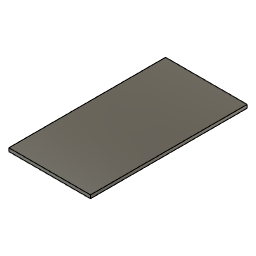
ionicthrusterassembly v7 (Autodesk Fusion 360 archive; units mm, degrees)
design "test"
Autodesk Fusion 360 part; units mm, degrees
(part 1 of 2)
sketch "Sketch1" plane through (0, 0, 0) normal (0, 0, 1) x (1, 0, 0)
  line L0 (0, 0) -> (125, 0)
  line L1 (125, 0) -> (125, 240)
  line L2 (125, 240) -> (0, 240)
  line L3 (0, 240) -> (0, 0)
  dimension "d1" = 125
  dimension "d2" = 240
  constraint horizontal L0
  constraint vertical L1
  constraint horizontal L2
  constraint vertical L3
  constraint coincident L0.start L3.end
  measures "d1" distance of L0.start L0.end
  measures "d2" distance of L0.start L2.end
extrude "Extrude1" add sketch "Sketch1" along normal blind 5

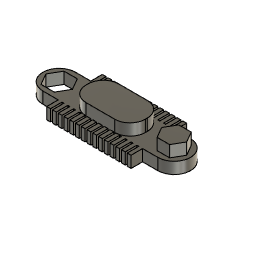
design "modularfingers"
Autodesk Fusion 360 part; units mm, degrees
sketch "Sketch1" plane through (0, 0, 0) normal (0, 0, 1) x (1, 0, 0)
  line L0 (0, -4.25) -> (30, -4.25)
  arc A0 (30, -4.25) -> (30, 4.25) centre (30, 0) ccw
  line L1 (30, 4.25) -> (0, 4.25)
  arc A1 (0, 4.25) -> (0, -4.25) centre (0, 0) ccw
  line L2 (0, 0) -> (30, 0) construction
  circle A2 centre (0, 0) radius 3 construction
  line L3 (-1.7321, 3) -> (-3.4641, 0)
  line L4 (-3.4641, 0) -> (-1.7321, -3)
  line L5 (-1.7321, -3) -> (1.7321, -3)
  line L6 (1.7321, -3) -> (3.4641, 0)
  line L7 (3.4641, 0) -> (1.7321, 3)
  line L8 (1.7321, 3) -> (-1.7321, 3)
  circle A3 centre (30, 0) radius 2.825 construction
  line L9 (33.262, 0) -> (31.631, 2.825)
  line L10 (31.631, 2.825) -> (28.369, 2.825)
  line L11 (28.369, 2.825) -> (26.738, 0)
  line L12 (26.738, 0) -> (28.369, -2.825)
  line L13 (28.369, -2.825) -> (31.631, -2.825)
  line L14 (31.631, -2.825) -> (33.262, 0)
  line L15 (18.738, -4.25) -> (11.262, -4.25)
  line L16 (7.262, -0.25) -> (7.262, 0.25)
  line L17 (11.262, 4.25) -> (18.738, 4.25)
  line L18 (22.738, 0.25) -> (22.738, -0.25)
  line L19 (22.738, -4.25) -> (7.262, 4.25) construction
  line L20 (7.262, -4.25) -> (22.738, 4.25) construction
  arc A4 (11.262, 4.25) -> (7.262, 0.25) centre (11.262, 0.25) ccw
  arc A5 (7.262, -0.25) -> (11.262, -4.25) centre (11.262, -0.25) ccw
  arc A6 (18.738, -4.25) -> (22.738, -0.25) centre (18.738, -0.25) ccw
  arc A7 (22.738, 0.25) -> (18.738, 4.25) centre (18.738, 0.25) ccw
  point P0 (30, 0)
  point P1 (15, 0)
  dimension "d1" = 30
  dimension "d2" = 4.25
  dimension "d14" = 60
  dimension "d15" = 5.65
  dimension "d16" = 6
  dimension "d17" = 60
  dimension "d18" = 4
  dimension "d19" = 4
  constraint tangent L0 A0
  constraint tangent A0 L1
  constraint parallel L0 L1
  constraint tangent L1 A1
  constraint tangent L0 A1
  constraint horizontal L2
  constraint coincident A1.centre L2.start
  constraint concentric A1 A2
  constraint concentric A0 A3
  constraint coincident P0 A0.centre
  constraint tangent A3 L9
  constraint tangent A2 L7
  constraint horizontal L15
  constraint perpendicular L15 L16
  constraint parallel L15 L17
  constraint parallel L16 L18
  constraint coincident L19 P1
  constraint coincident L20 P1
  constraint coincident L0 L19.start
  constraint midpoint L2 P1
  constraint coincident L19.end L16
  constraint coincident L19.end L17
  constraint tangent L16 A4
  constraint tangent L17 A4
  constraint coincident L20.start L16
  constraint coincident L20.start L15
  constraint tangent L16 A5
  constraint tangent L15 A5
  constraint equal A4 A5
  constraint coincident L19.start L18
  constraint coincident L19.start L15
  constraint tangent L18 A6
  constraint tangent L15 A6
  constraint equal A4 A6
  constraint coincident L20.end L18
  constraint coincident L20.end L17
  constraint tangent L18 A7
  constraint tangent L17 A7
  constraint equal A4 A7
  measures "d1" distance of A0.end L1.end
  measures "d2" radius of A0
  measures "d14" angle of L2 L7
  measures "d15" diameter of A3
  measures "d16" diameter of A2
  measures "d17" angle of L2 L14
  measures "d18" distance of L11.end L18
  measures "d19" radius of A4
extrude "Extrude1" add sketch "Sketch1" along normal blind 3 contours L0 L1 A1 L16 A4 A5 | L0 A0 L1 L18 A6 A7 makes body 1 at (4.2732, -1.6372, 0) makes body 2 at (25.8943, 1.4006, 0)
extrude "Extrude3" add sketch "Sketch1" along normal blind 6 contours L0 L1 L15 L16 L17 L18 A4 A5 A6 A7 | L9 L10 L11 L12 L13 L14 bodies 1 2
sketch "Sketch3" plane through (0, -4.25, 0) normal (0, -1, 0) x (1, 0, 0)
  line L0 (0, 0) -> (30, 0)
  line L1 (30, 0) -> (30, 3)
  line L2 (30, 3) -> (18.738, 3)
  line L3 (18.738, 3) -> (18.738, 6)
  line L4 (18.738, 6) -> (11.262, 6)
  line L5 (11.262, 6) -> (11.262, 3)
  line L6 (11.262, 3) -> (0, 3)
  line L7 (0, 3) -> (0, 0)
  line L8 (4, 3) -> (5, 3)
  line L9 (5, 3) -> (5, 0)
  line L10 (5, 0) -> (4, 0)
  line L11 (4, 0) -> (4, 3)
  line L12 (6.5, 3) -> (6.5, 0)
  line L13 (5.5, 3) -> (6.5, 3)
  line L14 (5.5, 0) -> (5.5, 3)
  line L15 (6.5, 0) -> (5.5, 0)
  line L16 (8, 3) -> (8, 0)
  line L17 (7, 3) -> (8, 3)
  line L18 (7, 0) -> (7, 3)
  line L19 (8, 0) -> (7, 0)
  line L20 (9.5, 3) -> (9.5, 0)
  line L21 (8.5, 3) -> (9.5, 3)
  line L22 (8.5, 0) -> (8.5, 3)
  line L23 (9.5, 0) -> (8.5, 0)
  line L24 (11, 3) -> (11, 0)
  line L25 (10, 3) -> (11, 3)
  line L26 (10, 0) -> (10, 3)
  line L27 (11, 0) -> (10, 0)
  line L28 (12.5, 3) -> (12.5, 0)
  line L29 (11.5, 3) -> (12.5, 3)
  line L30 (11.5, 0) -> (11.5, 3)
  line L31 (12.5, 0) -> (11.5, 0)
  line L32 (14, 3) -> (14, 0)
  line L33 (13, 3) -> (14, 3)
  line L34 (13, 0) -> (13, 3)
  line L35 (14, 0) -> (13, 0)
  line L36 (15.5, 3) -> (15.5, 0)
  line L37 (14.5, 3) -> (15.5, 3)
  line L38 (14.5, 0) -> (14.5, 3)
  line L39 (15.5, 0) -> (14.5, 0)
  line L40 (17, 3) -> (17, 0)
  line L41 (16, 3) -> (17, 3)
  line L42 (16, 0) -> (16, 3)
  line L43 (17, 0) -> (16, 0)
  line L44 (18.5, 3) -> (18.5, 0)
  line L45 (17.5, 3) -> (18.5, 3)
  line L46 (17.5, 0) -> (17.5, 3)
  line L47 (18.5, 0) -> (17.5, 0)
  line L48 (20, 3) -> (20, 0)
  line L49 (19, 3) -> (20, 3)
  line L50 (19, 0) -> (19, 3)
  line L51 (20, 0) -> (19, 0)
  line L52 (21.5, 3) -> (21.5, 0)
  line L53 (20.5, 3) -> (21.5, 3)
  line L54 (20.5, 0) -> (20.5, 3)
  line L55 (21.5, 0) -> (20.5, 0)
  line L56 (23, 3) -> (23, 0)
  line L57 (22, 3) -> (23, 3)
  line L58 (22, 0) -> (22, 3)
  line L59 (23, 0) -> (22, 0)
  line L60 (24.5, 3) -> (24.5, 0)
  line L61 (23.5, 3) -> (24.5, 3)
  line L62 (23.5, 0) -> (23.5, 3)
  line L63 (24.5, 0) -> (23.5, 0)
  line L64 (26, 3) -> (26, 0)
  line L65 (25, 3) -> (26, 3)
  line L66 (25, 0) -> (25, 3)
  line L67 (26, 0) -> (25, 0)
  dimension "d39" = 1
  dimension "d40" = 4
  dimension "d47" = 21
  dimension "d48" = 0
  constraint horizontal L8
  constraint vertical L9
  constraint horizontal L10
  constraint vertical L11
  constraint coincident L0 L9.end
  constraint coincident L6 L8.start
  measures "d39" distance of L9.end L10.end
  measures "d40" distance of L7 L11
extrude "Extrude5" add sketch "Sketch3" along normal blind 3 contours L0 L6 L8 L9 L10 L11 | L0 L6 L12 L13 L14 L15 | L0 L6 L16 L17 L18 L19 | L0 L6 L20 L21 L22 L23 | L0 L6 L24 L25 L26 L27 | L0 L28 L29 L30 L31 | L0 L32 L33 L34 L35 | L0 L36 L37 L38 L39 | L0 L2 L48 L49 L50 L51 | L0 L40 L41 L42 L43 | L0 L2 L52 L53 L54 L55 | L0 L44 L45 L46 L47 | L0 L2 L56 L57 L58 L59 | L0 L2 L60 L61 L62 L63 | L0 L2 L64 L65 L66 L67 bodies 1
ref_plane "WorkPlane2" through (28, 0, 1.5) normal (0, -1, 0) x (1, 0, 0)
mirror "Mirror2" about plane through (28, 0, 1.5) normal (0, -1, 0) of bodies 1 merged
equation "d1 = length"
equation "d2 = arc_Length"
equation "height = 6 mm"
equation "length = 30 mm"
equation "total_length = 30 mm + 8.5 mm"
equation "arc_Length = ( total_length - length ) / 2"
equation "DegreePolygon = ( 360 / 6 ) * 1 deg"
equation "Polygon_Length = 6 mm"
equation "NPolygonSides = 6"
equation "d14 = DegreePolygon"
equation "d15 = Polygon_Length - Hole_OFFSET"
equation "d16 = Polygon_Length"
equation "d17 = DegreePolygon"
equation "d18 = offsetdistance"
equation "d19 = arc_Polygon"
equation "arc_Polygon = 4 mm"
equation "offsetdistance = 4 mm"
equation "d22 = ( height / 2 mm ) * 1 mm"
equation "d26 = height"
equation "Hole_OFFSET = 0.35 mm"
equation "d39 = pattounes_width"
equation "d40 = pattounes_offset"
equation "pattounes_offset = 4 mm"
equation "pattounes_width = 1 mm"
equation "NPattounes = 15"
equation "d45 = NPattounes"
equation "d47 = length - pattounes_offset * 2 - pattounes_width"
equation "d51 = -arc_Length"

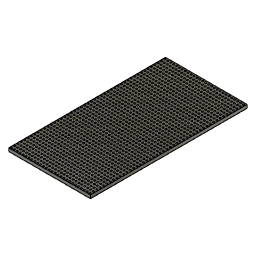
design "base"
Autodesk Fusion 360 part; units mm, degrees
sketch "Sketch1" plane through (0, 0, 0) normal (0, 0, 1) x (1, 0, 0)
  line L0 (0, 0) -> (125, 0)
  line L1 (125, 0) -> (125, 240)
  line L2 (125, 240) -> (0, 240)
  line L3 (0, 240) -> (0, 0)
  line L4 (0, 0) -> (2, 0) construction
  line L5 (2, 0) -> (2, 2) construction
  line L6 (2, 2) -> (0, 2) construction
  line L7 (0, 2) -> (0, 0) construction
  circle A0 centre (2, 2) radius 1.25
  circle A1 centre (6.4643, 2) radius 1.25
  circle A2 centre (10.9286, 2) radius 1.25
  circle A3 centre (15.3929, 2) radius 1.25
  circle A4 centre (19.8571, 2) radius 1.25
  circle A5 centre (24.3214, 2) radius 1.25
  circle A6 centre (28.7857, 2) radius 1.25
  circle A7 centre (33.25, 2) radius 1.25
  circle A8 centre (37.7143, 2) radius 1.25
  circle A9 centre (2, 7.1064) radius 1.25
  circle A10 centre (6.4643, 7.1064) radius 1.25
  circle A11 centre (10.9286, 7.1064) radius 1.25
  circle A12 centre (15.3929, 7.1064) radius 1.25
  circle A13 centre (19.8571, 7.1064) radius 1.25
  circle A14 centre (24.3214, 7.1064) radius 1.25
  circle A15 centre (28.7857, 7.1064) radius 1.25
  circle A16 centre (33.25, 7.1064) radius 1.25
  circle A17 centre (37.7143, 7.1064) radius 1.25
  circle A18 centre (2, 12.2128) radius 1.25
  circle A19 centre (6.4643, 12.2128) radius 1.25
  circle A20 centre (10.9286, 12.2128) radius 1.25
  circle A21 centre (15.3929, 12.2128) radius 1.25
  circle A22 centre (19.8571, 12.2128) radius 1.25
  circle A23 centre (24.3214, 12.2128) radius 1.25
  circle A24 centre (28.7857, 12.2128) radius 1.25
  circle A25 centre (33.25, 12.2128) radius 1.25
  circle A26 centre (37.7143, 12.2128) radius 1.25
  circle A27 centre (2, 17.3191) radius 1.25
  circle A28 centre (6.4643, 17.3191) radius 1.25
  circle A29 centre (10.9286, 17.3191) radius 1.25
  circle A30 centre (15.3929, 17.3191) radius 1.25
  circle A31 centre (19.8571, 17.3191) radius 1.25
  circle A32 centre (24.3214, 17.3191) radius 1.25
  circle A33 centre (28.7857, 17.3191) radius 1.25
  circle A34 centre (33.25, 17.3191) radius 1.25
  circle A35 centre (37.7143, 17.3191) radius 1.25
  circle A36 centre (2, 22.4255) radius 1.25
  circle A37 centre (6.4643, 22.4255) radius 1.25
  circle A38 centre (10.9286, 22.4255) radius 1.25
  circle A39 centre (15.3929, 22.4255) radius 1.25
  circle A40 centre (19.8571, 22.4255) radius 1.25
  circle A41 centre (24.3214, 22.4255) radius 1.25
  circle A42 centre (28.7857, 22.4255) radius 1.25
  circle A43 centre (33.25, 22.4255) radius 1.25
  circle A44 centre (37.7143, 22.4255) radius 1.25
  circle A45 centre (2, 27.5319) radius 1.25
  circle A46 centre (6.4643, 27.5319) radius 1.25
  circle A47 centre (10.9286, 27.5319) radius 1.25
  circle A48 centre (15.3929, 27.5319) radius 1.25
  circle A49 centre (19.8571, 27.5319) radius 1.25
  circle A50 centre (24.3214, 27.5319) radius 1.25
  circle A51 centre (28.7857, 27.5319) radius 1.25
  circle A52 centre (33.25, 27.5319) radius 1.25
  circle A53 centre (37.7143, 27.5319) radius 1.25
  circle A54 centre (2, 32.6383) radius 1.25
  circle A55 centre (6.4643, 32.6383) radius 1.25
  circle A56 centre (10.9286, 32.6383) radius 1.25
  circle A57 centre (15.3929, 32.6383) radius 1.25
  circle A58 centre (19.8571, 32.6383) radius 1.25
  circle A59 centre (24.3214, 32.6383) radius 1.25
  circle A60 centre (28.7857, 32.6383) radius 1.25
  circle A61 centre (33.25, 32.6383) radius 1.25
  circle A62 centre (37.7143, 32.6383) radius 1.25
  circle A63 centre (2, 37.7447) radius 1.25
  circle A64 centre (6.4643, 37.7447) radius 1.25
  circle A65 centre (10.9286, 37.7447) radius 1.25
  circle A66 centre (15.3929, 37.7447) radius 1.25
  circle A67 centre (19.8571, 37.7447) radius 1.25
  circle A68 centre (24.3214, 37.7447) radius 1.25
  circle A69 centre (28.7857, 37.7447) radius 1.25
  circle A70 centre (33.25, 37.7447) radius 1.25
  circle A71 centre (37.7143, 37.7447) radius 1.25
  circle A72 centre (2, 42.8511) radius 1.25
  circle A73 centre (6.4643, 42.8511) radius 1.25
  circle A74 centre (10.9286, 42.8511) radius 1.25
  circle A75 centre (15.3929, 42.8511) radius 1.25
  circle A76 centre (19.8571, 42.8511) radius 1.25
  circle A77 centre (24.3214, 42.8511) radius 1.25
  circle A78 centre (28.7857, 42.8511) radius 1.25
  circle A79 centre (33.25, 42.8511) radius 1.25
  circle A80 centre (37.7143, 42.8511) radius 1.25
  circle A81 centre (2, 47.9574) radius 1.25
  circle A82 centre (6.4643, 47.9574) radius 1.25
  circle A83 centre (10.9286, 47.9574) radius 1.25
  circle A84 centre (15.3929, 47.9574) radius 1.25
  circle A85 centre (19.8571, 47.9574) radius 1.25
  circle A86 centre (24.3214, 47.9574) radius 1.25
  circle A87 centre (28.7857, 47.9574) radius 1.25
  circle A88 centre (33.25, 47.9574) radius 1.25
  circle A89 centre (37.7143, 47.9574) radius 1.25
  circle A90 centre (2, 53.0638) radius 1.25
  circle A91 centre (6.4643, 53.0638) radius 1.25
  circle A92 centre (10.9286, 53.0638) radius 1.25
  circle A93 centre (15.3929, 53.0638) radius 1.25
  circle A94 centre (19.8571, 53.0638) radius 1.25
  circle A95 centre (24.3214, 53.0638) radius 1.25
  circle A96 centre (28.7857, 53.0638) radius 1.25
  circle A97 centre (33.25, 53.0638) radius 1.25
  circle A98 centre (37.7143, 53.0638) radius 1.25
  circle A99 centre (2, 58.1702) radius 1.25
  circle A100 centre (6.4643, 58.1702) radius 1.25
  circle A101 centre (10.9286, 58.1702) radius 1.25
  circle A102 centre (15.3929, 58.1702) radius 1.25
  circle A103 centre (19.8571, 58.1702) radius 1.25
  circle A104 centre (24.3214, 58.1702) radius 1.25
  circle A105 centre (28.7857, 58.1702) radius 1.25
  circle A106 centre (33.25, 58.1702) radius 1.25
  circle A107 centre (37.7143, 58.1702) radius 1.25
  circle A108 centre (2, 63.2766) radius 1.25
  circle A109 centre (6.4643, 63.2766) radius 1.25
  circle A110 centre (10.9286, 63.2766) radius 1.25
  circle A111 centre (15.3929, 63.2766) radius 1.25
  circle A112 centre (19.8571, 63.2766) radius 1.25
  circle A113 centre (24.3214, 63.2766) radius 1.25
  circle A114 centre (28.7857, 63.2766) radius 1.25
  circle A115 centre (33.25, 63.2766) radius 1.25
  circle A116 centre (37.7143, 63.2766) radius 1.25
  circle A117 centre (2, 68.383) radius 1.25
  circle A118 centre (6.4643, 68.383) radius 1.25
  circle A119 centre (10.9286, 68.383) radius 1.25
  circle A120 centre (15.3929, 68.383) radius 1.25
  circle A121 centre (19.8571, 68.383) radius 1.25
  circle A122 centre (24.3214, 68.383) radius 1.25
  circle A123 centre (28.7857, 68.383) radius 1.25
  circle A124 centre (33.25, 68.383) radius 1.25
  circle A125 centre (37.7143, 68.383) radius 1.25
  circle A126 centre (2, 73.4894) radius 1.25
  circle A127 centre (6.4643, 73.4894) radius 1.25
  circle A128 centre (10.9286, 73.4894) radius 1.25
  circle A129 centre (15.3929, 73.4894) radius 1.25
  circle A130 centre (19.8571, 73.4894) radius 1.25
  circle A131 centre (24.3214, 73.4894) radius 1.25
  circle A132 centre (28.7857, 73.4894) radius 1.25
  circle A133 centre (33.25, 73.4894) radius 1.25
  circle A134 centre (37.7143, 73.4894) radius 1.25
  circle A135 centre (2, 78.5957) radius 1.25
  circle A136 centre (6.4643, 78.5957) radius 1.25
  circle A137 centre (10.9286, 78.5957) radius 1.25
  circle A138 centre (15.3929, 78.5957) radius 1.25
  circle A139 centre (19.8571, 78.5957) radius 1.25
  circle A140 centre (24.3214, 78.5957) radius 1.25
  circle A141 centre (28.7857, 78.5957) radius 1.25
  circle A142 centre (33.25, 78.5957) radius 1.25
  circle A143 centre (37.7143, 78.5957) radius 1.25
  circle A144 centre (2, 83.7021) radius 1.25
  circle A145 centre (6.4643, 83.7021) radius 1.25
  circle A146 centre (10.9286, 83.7021) radius 1.25
  circle A147 centre (15.3929, 83.7021) radius 1.25
  circle A148 centre (19.8571, 83.7021) radius 1.25
  circle A149 centre (24.3214, 83.7021) radius 1.25
  circle A150 centre (28.7857, 83.7021) radius 1.25
  circle A151 centre (33.25, 83.7021) radius 1.25
  circle A152 centre (37.7143, 83.7021) radius 1.25
  circle A153 centre (2, 88.8085) radius 1.25
  circle A154 centre (6.4643, 88.8085) radius 1.25
  circle A155 centre (10.9286, 88.8085) radius 1.25
  circle A156 centre (15.3929, 88.8085) radius 1.25
  circle A157 centre (19.8571, 88.8085) radius 1.25
  circle A158 centre (24.3214, 88.8085) radius 1.25
  circle A159 centre (28.7857, 88.8085) radius 1.25
  circle A160 centre (33.25, 88.8085) radius 1.25
  circle A161 centre (37.7143, 88.8085) radius 1.25
  circle A162 centre (2, 93.9149) radius 1.25
  circle A163 centre (6.4643, 93.9149) radius 1.25
  circle A164 centre (10.9286, 93.9149) radius 1.25
  circle A165 centre (15.3929, 93.9149) radius 1.25
  circle A166 centre (19.8571, 93.9149) radius 1.25
  circle A167 centre (24.3214, 93.9149) radius 1.25
  circle A168 centre (28.7857, 93.9149) radius 1.25
  circle A169 centre (33.25, 93.9149) radius 1.25
  circle A170 centre (37.7143, 93.9149) radius 1.25
  circle A171 centre (2, 99.0213) radius 1.25
  circle A172 centre (6.4643, 99.0213) radius 1.25
  circle A173 centre (10.9286, 99.0213) radius 1.25
  circle A174 centre (15.3929, 99.0213) radius 1.25
  circle A175 centre (19.8571, 99.0213) radius 1.25
  circle A176 centre (24.3214, 99.0213) radius 1.25
  circle A177 centre (28.7857, 99.0213) radius 1.25
  circle A178 centre (33.25, 99.0213) radius 1.25
  circle A179 centre (37.7143, 99.0213) radius 1.25
  circle A180 centre (2, 104.1277) radius 1.25
  circle A181 centre (6.4643, 104.1277) radius 1.25
  circle A182 centre (10.9286, 104.1277) radius 1.25
  circle A183 centre (15.3929, 104.1277) radius 1.25
  circle A184 centre (19.8571, 104.1277) radius 1.25
  circle A185 centre (24.3214, 104.1277) radius 1.25
  circle A186 centre (28.7857, 104.1277) radius 1.25
  circle A187 centre (33.25, 104.1277) radius 1.25
  circle A188 centre (37.7143, 104.1277) radius 1.25
  circle A189 centre (2, 109.234) radius 1.25
  circle A190 centre (6.4643, 109.234) radius 1.25
  circle A191 centre (10.9286, 109.234) radius 1.25
  circle A192 centre (15.3929, 109.234) radius 1.25
  circle A193 centre (19.8571, 109.234) radius 1.25
  circle A194 centre (24.3214, 109.234) radius 1.25
  circle A195 centre (28.7857, 109.234) radius 1.25
  circle A196 centre (33.25, 109.234) radius 1.25
  circle A197 centre (37.7143, 109.234) radius 1.25
  circle A198 centre (2, 114.3404) radius 1.25
  circle A199 centre (6.4643, 114.3404) radius 1.25
  circle A200 centre (10.9286, 114.3404) radius 1.25
  circle A201 centre (15.3929, 114.3404) radius 1.25
  circle A202 centre (19.8571, 114.3404) radius 1.25
  circle A203 centre (24.3214, 114.3404) radius 1.25
  circle A204 centre (28.7857, 114.3404) radius 1.25
  circle A205 centre (33.25, 114.3404) radius 1.25
  circle A206 centre (37.7143, 114.3404) radius 1.25
  circle A207 centre (2, 119.4468) radius 1.25
  circle A208 centre (6.4643, 119.4468) radius 1.25
  circle A209 centre (10.9286, 119.4468) radius 1.25
  circle A210 centre (15.3929, 119.4468) radius 1.25
  circle A211 centre (19.8571, 119.4468) radius 1.25
  circle A212 centre (24.3214, 119.4468) radius 1.25
  circle A213 centre (28.7857, 119.4468) radius 1.25
  circle A214 centre (33.25, 119.4468) radius 1.25
  circle A215 centre (37.7143, 119.4468) radius 1.25
  circle A216 centre (2, 124.5532) radius 1.25
  circle A217 centre (6.4643, 124.5532) radius 1.25
  circle A218 centre (10.9286, 124.5532) radius 1.25
  circle A219 centre (15.3929, 124.5532) radius 1.25
  circle A220 centre (19.8571, 124.5532) radius 1.25
  circle A221 centre (24.3214, 124.5532) radius 1.25
  circle A222 centre (28.7857, 124.5532) radius 1.25
  circle A223 centre (33.25, 124.5532) radius 1.25
  circle A224 centre (37.7143, 124.5532) radius 1.25
  circle A225 centre (2, 129.6596) radius 1.25
  circle A226 centre (6.4643, 129.6596) radius 1.25
  circle A227 centre (10.9286, 129.6596) radius 1.25
  circle A228 centre (15.3929, 129.6596) radius 1.25
  circle A229 centre (19.8571, 129.6596) radius 1.25
  circle A230 centre (24.3214, 129.6596) radius 1.25
  circle A231 centre (28.7857, 129.6596) radius 1.25
  circle A232 centre (33.25, 129.6596) radius 1.25
  circle A233 centre (37.7143, 129.6596) radius 1.25
  circle A234 centre (2, 134.766) radius 1.25
  circle A235 centre (6.4643, 134.766) radius 1.25
  circle A236 centre (10.9286, 134.766) radius 1.25
  circle A237 centre (15.3929, 134.766) radius 1.25
  circle A238 centre (19.8571, 134.766) radius 1.25
  circle A239 centre (24.3214, 134.766) radius 1.25
  circle A240 centre (28.7857, 134.766) radius 1.25
  circle A241 centre (33.25, 134.766) radius 1.25
  circle A242 centre (37.7143, 134.766) radius 1.25
  circle A243 centre (2, 139.8723) radius 1.25
  circle A244 centre (6.4643, 139.8723) radius 1.25
  circle A245 centre (10.9286, 139.8723) radius 1.25
  circle A246 centre (15.3929, 139.8723) radius 1.25
  circle A247 centre (19.8571, 139.8723) radius 1.25
  circle A248 centre (24.3214, 139.8723) radius 1.25
  circle A249 centre (28.7857, 139.8723) radius 1.25
  circle A250 centre (33.25, 139.8723) radius 1.25
  circle A251 centre (37.7143, 139.8723) radius 1.25
  circle A252 centre (2, 144.9787) radius 1.25
  circle A253 centre (6.4643, 144.9787) radius 1.25
  circle A254 centre (10.9286, 144.9787) radius 1.25
  circle A255 centre (15.3929, 144.9787) radius 1.25
  circle A256 centre (19.8571, 144.9787) radius 1.25
  circle A257 centre (24.3214, 144.9787) radius 1.25
  circle A258 centre (28.7857, 144.9787) radius 1.25
  circle A259 centre (33.25, 144.9787) radius 1.25
  circle A260 centre (37.7143, 144.9787) radius 1.25
  circle A261 centre (2, 150.0851) radius 1.25
  circle A262 centre (6.4643, 150.0851) radius 1.25
  circle A263 centre (10.9286, 150.0851) radius 1.25
  circle A264 centre (15.3929, 150.0851) radius 1.25
  circle A265 centre (19.8571, 150.0851) radius 1.25
  circle A266 centre (24.3214, 150.0851) radius 1.25
  circle A267 centre (28.7857, 150.0851) radius 1.25
  circle A268 centre (33.25, 150.0851) radius 1.25
  circle A269 centre (37.7143, 150.0851) radius 1.25
  circle A270 centre (2, 155.1915) radius 1.25
  circle A271 centre (6.4643, 155.1915) radius 1.25
  circle A272 centre (10.9286, 155.1915) radius 1.25
  circle A273 centre (15.3929, 155.1915) radius 1.25
  circle A274 centre (19.8571, 155.1915) radius 1.25
  circle A275 centre (24.3214, 155.1915) radius 1.25
  circle A276 centre (28.7857, 155.1915) radius 1.25
  circle A277 centre (33.25, 155.1915) radius 1.25
  circle A278 centre (37.7143, 155.1915) radius 1.25
  circle A279 centre (2, 160.2979) radius 1.25
  circle A280 centre (6.4643, 160.2979) radius 1.25
  circle A281 centre (10.9286, 160.2979) radius 1.25
  circle A282 centre (15.3929, 160.2979) radius 1.25
  circle A283 centre (19.8571, 160.2979) radius 1.25
  circle A284 centre (24.3214, 160.2979) radius 1.25
  circle A285 centre (28.7857, 160.2979) radius 1.25
  circle A286 centre (33.25, 160.2979) radius 1.25
  circle A287 centre (37.7143, 160.2979) radius 1.25
  circle A288 centre (2, 165.4043) radius 1.25
  circle A289 centre (6.4643, 165.4043) radius 1.25
  circle A290 centre (10.9286, 165.4043) radius 1.25
  circle A291 centre (15.3929, 165.4043) radius 1.25
  circle A292 centre (19.8571, 165.4043) radius 1.25
  circle A293 centre (24.3214, 165.4043) radius 1.25
  circle A294 centre (28.7857, 165.4043) radius 1.25
  circle A295 centre (33.25, 165.4043) radius 1.25
  circle A296 centre (37.7143, 165.4043) radius 1.25
  circle A297 centre (2, 170.5106) radius 1.25
  circle A298 centre (6.4643, 170.5106) radius 1.25
  circle A299 centre (10.9286, 170.5106) radius 1.25
  circle A300 centre (15.3929, 170.5106) radius 1.25
  circle A301 centre (19.8571, 170.5106) radius 1.25
  circle A302 centre (24.3214, 170.5106) radius 1.25
  circle A303 centre (28.7857, 170.5106) radius 1.25
  circle A304 centre (33.25, 170.5106) radius 1.25
  circle A305 centre (37.7143, 170.5106) radius 1.25
  circle A306 centre (2, 175.617) radius 1.25
  circle A307 centre (6.4643, 175.617) radius 1.25
  circle A308 centre (10.9286, 175.617) radius 1.25
  circle A309 centre (15.3929, 175.617) radius 1.25
  circle A310 centre (19.8571, 175.617) radius 1.25
  circle A311 centre (24.3214, 175.617) radius 1.25
  circle A312 centre (28.7857, 175.617) radius 1.25
  circle A313 centre (33.25, 175.617) radius 1.25
  circle A314 centre (37.7143, 175.617) radius 1.25
  circle A315 centre (2, 180.7234) radius 1.25
  circle A316 centre (6.4643, 180.7234) radius 1.25
  circle A317 centre (10.9286, 180.7234) radius 1.25
  circle A318 centre (15.3929, 180.7234) radius 1.25
  circle A319 centre (19.8571, 180.7234) radius 1.25
  circle A320 centre (24.3214, 180.7234) radius 1.25
  circle A321 centre (28.7857, 180.7234) radius 1.25
  circle A322 centre (33.25, 180.7234) radius 1.25
  circle A323 centre (37.7143, 180.7234) radius 1.25
  circle A324 centre (2, 185.8298) radius 1.25
  circle A325 centre (6.4643, 185.8298) radius 1.25
  circle A326 centre (10.9286, 185.8298) radius 1.25
  circle A327 centre (15.3929, 185.8298) radius 1.25
  circle A328 centre (19.8571, 185.8298) radius 1.25
  circle A329 centre (24.3214, 185.8298) radius 1.25
  circle A330 centre (28.7857, 185.8298) radius 1.25
  circle A331 centre (33.25, 185.8298) radius 1.25
  circle A332 centre (37.7143, 185.8298) radius 1.25
  circle A333 centre (2, 190.9362) radius 1.25
  circle A334 centre (6.4643, 190.9362) radius 1.25
  circle A335 centre (10.9286, 190.9362) radius 1.25
  circle A336 centre (15.3929, 190.9362) radius 1.25
  circle A337 centre (19.8571, 190.9362) radius 1.25
  circle A338 centre (24.3214, 190.9362) radius 1.25
  circle A339 centre (28.7857, 190.9362) radius 1.25
  circle A340 centre (33.25, 190.9362) radius 1.25
  circle A341 centre (37.7143, 190.9362) radius 1.25
  circle A342 centre (2, 196.0426) radius 1.25
  circle A343 centre (6.4643, 196.0426) radius 1.25
  circle A344 centre (10.9286, 196.0426) radius 1.25
  circle A345 centre (15.3929, 196.0426) radius 1.25
  circle A346 centre (19.8571, 196.0426) radius 1.25
  circle A347 centre (24.3214, 196.0426) radius 1.25
  circle A348 centre (28.7857, 196.0426) radius 1.25
  circle A349 centre (33.25, 196.0426) radius 1.25
  circle A350 centre (37.7143, 196.0426) radius 1.25
  circle A351 centre (2, 201.1489) radius 1.25
  circle A352 centre (6.4643, 201.1489) radius 1.25
  circle A353 centre (10.9286, 201.1489) radius 1.25
  circle A354 centre (15.3929, 201.1489) radius 1.25
  circle A355 centre (19.8571, 201.1489) radius 1.25
  circle A356 centre (24.3214, 201.1489) radius 1.25
  circle A357 centre (28.7857, 201.1489) radius 1.25
  circle A358 centre (33.25, 201.1489) radius 1.25
  circle A359 centre (37.7143, 201.1489) radius 1.25
  circle A360 centre (2, 206.2553) radius 1.25
  circle A361 centre (6.4643, 206.2553) radius 1.25
  circle A362 centre (10.9286, 206.2553) radius 1.25
  circle A363 centre (15.3929, 206.2553) radius 1.25
  circle A364 centre (19.8571, 206.2553) radius 1.25
  circle A365 centre (24.3214, 206.2553) radius 1.25
  circle A366 centre (28.7857, 206.2553) radius 1.25
  circle A367 centre (33.25, 206.2553) radius 1.25
  circle A368 centre (37.7143, 206.2553) radius 1.25
  circle A369 centre (2, 211.3617) radius 1.25
  circle A370 centre (6.4643, 211.3617) radius 1.25
  circle A371 centre (10.9286, 211.3617) radius 1.25
  circle A372 centre (15.3929, 211.3617) radius 1.25
  circle A373 centre (19.8571, 211.3617) radius 1.25
  circle A374 centre (24.3214, 211.3617) radius 1.25
  circle A375 centre (28.7857, 211.3617) radius 1.25
  circle A376 centre (33.25, 211.3617) radius 1.25
  circle A377 centre (37.7143, 211.3617) radius 1.25
  circle A378 centre (2, 216.4681) radius 1.25
  circle A379 centre (6.4643, 216.4681) radius 1.25
  circle A380 centre (10.9286, 216.4681) radius 1.25
  circle A381 centre (15.3929, 216.4681) radius 1.25
  circle A382 centre (19.8571, 216.4681) radius 1.25
  circle A383 centre (24.3214, 216.4681) radius 1.25
  circle A384 centre (28.7857, 216.4681) radius 1.25
  circle A385 centre (33.25, 216.4681) radius 1.25
  circle A386 centre (37.7143, 216.4681) radius 1.25
  circle A387 centre (2, 221.5745) radius 1.25
  circle A388 centre (6.4643, 221.5745) radius 1.25
  circle A389 centre (10.9286, 221.5745) radius 1.25
  circle A390 centre (15.3929, 221.5745) radius 1.25
  circle A391 centre (19.8571, 221.5745) radius 1.25
  circle A392 centre (24.3214, 221.5745) radius 1.25
  circle A393 centre (28.7857, 221.5745) radius 1.25
  circle A394 centre (33.25, 221.5745) radius 1.25
  circle A395 centre (37.7143, 221.5745) radius 1.25
  circle A396 centre (2, 226.6809) radius 1.25
  circle A397 centre (6.4643, 226.6809) radius 1.25
  circle A398 centre (10.9286, 226.6809) radius 1.25
  circle A399 centre (15.3929, 226.6809) radius 1.25
  circle A400 centre (19.8571, 226.6809) radius 1.25
  circle A401 centre (24.3214, 226.6809) radius 1.25
  circle A402 centre (28.7857, 226.6809) radius 1.25
  circle A403 centre (33.25, 226.6809) radius 1.25
  circle A404 centre (37.7143, 226.6809) radius 1.25
  circle A405 centre (2, 231.7872) radius 1.25
  circle A406 centre (6.4643, 231.7872) radius 1.25
  circle A407 centre (10.9286, 231.7872) radius 1.25
  circle A408 centre (15.3929, 231.7872) radius 1.25
  circle A409 centre (19.8571, 231.7872) radius 1.25
  circle A410 centre (24.3214, 231.7872) radius 1.25
  circle A411 centre (28.7857, 231.7872) radius 1.25
  circle A412 centre (33.25, 231.7872) radius 1.25
  circle A413 centre (37.7143, 231.7872) radius 1.25
  circle A414 centre (2, 236.8936) radius 1.25
  circle A415 centre (6.4643, 236.8936) radius 1.25
  circle A416 centre (10.9286, 236.8936) radius 1.25
  circle A417 centre (15.3929, 236.8936) radius 1.25
  circle A418 centre (19.8571, 236.8936) radius 1.25
  circle A419 centre (24.3214, 236.8936) radius 1.25
  circle A420 centre (28.7857, 236.8936) radius 1.25
  circle A421 centre (33.25, 236.8936) radius 1.25
  circle A422 centre (37.7143, 236.8936) radius 1.25
  circle A423 centre (2, 242) radius 1.25
  circle A424 centre (6.4643, 242) radius 1.25
  circle A425 centre (10.9286, 242) radius 1.25
  circle A426 centre (15.3929, 242) radius 1.25
  circle A427 centre (19.8571, 242) radius 1.25
  circle A428 centre (24.3214, 242) radius 1.25
  circle A429 centre (28.7857, 242) radius 1.25
  circle A430 centre (33.25, 242) radius 1.25
  circle A431 centre (37.7143, 242) radius 1.25
  circle A432 centre (42.1786, 2) radius 1.25
  circle A433 centre (46.6429, 2) radius 1.25
  circle A434 centre (51.1071, 2) radius 1.25
  circle A435 centre (55.5714, 2) radius 1.25
  circle A436 centre (60.0357, 2) radius 1.25
  circle A437 centre (64.5, 2) radius 1.25
  circle A438 centre (68.9643, 2) radius 1.25
  circle A439 centre (73.4286, 2) radius 1.25
  circle A440 centre (77.8929, 2) radius 1.25
  circle A441 centre (82.3571, 2) radius 1.25
  circle A442 centre (86.8214, 2) radius 1.25
  circle A443 centre (91.2857, 2) radius 1.25
  circle A444 centre (95.75, 2) radius 1.25
  circle A445 centre (100.2143, 2) radius 1.25
  circle A446 centre (104.6786, 2) radius 1.25
  circle A447 centre (109.1429, 2) radius 1.25
  circle A448 centre (113.6071, 2) radius 1.25
  circle A449 centre (118.0714, 2) radius 1.25
  circle A450 centre (122.5357, 2) radius 1.25
  circle A451 centre (127, 2) radius 1.25
  circle A452 centre (42.1786, 7.1064) radius 1.25
  circle A453 centre (46.6429, 7.1064) radius 1.25
  circle A454 centre (51.1071, 7.1064) radius 1.25
  circle A455 centre (55.5714, 7.1064) radius 1.25
  circle A456 centre (60.0357, 7.1064) radius 1.25
  circle A457 centre (64.5, 7.1064) radius 1.25
  circle A458 centre (68.9643, 7.1064) radius 1.25
  circle A459 centre (73.4286, 7.1064) radius 1.25
  circle A460 centre (77.8929, 7.1064) radius 1.25
  circle A461 centre (82.3571, 7.1064) radius 1.25
  circle A462 centre (86.8214, 7.1064) radius 1.25
  circle A463 centre (91.2857, 7.1064) radius 1.25
  circle A464 centre (95.75, 7.1064) radius 1.25
  circle A465 centre (100.2143, 7.1064) radius 1.25
  circle A466 centre (104.6786, 7.1064) radius 1.25
  circle A467 centre (109.1429, 7.1064) radius 1.25
  circle A468 centre (113.6071, 7.1064) radius 1.25
  circle A469 centre (118.0714, 7.1064) radius 1.25
  circle A470 centre (122.5357, 7.1064) radius 1.25
  circle A471 centre (127, 7.1064) radius 1.25
  circle A472 centre (42.1786, 12.2128) radius 1.25
  circle A473 centre (46.6429, 12.2128) radius 1.25
  circle A474 centre (51.1071, 12.2128) radius 1.25
  circle A475 centre (55.5714, 12.2128) radius 1.25
  circle A476 centre (60.0357, 12.2128) radius 1.25
  circle A477 centre (64.5, 12.2128) radius 1.25
  circle A478 centre (68.9643, 12.2128) radius 1.25
  circle A479 centre (73.4286, 12.2128) radius 1.25
  circle A480 centre (77.8929, 12.2128) radius 1.25
  circle A481 centre (82.3571, 12.2128) radius 1.25
  circle A482 centre (86.8214, 12.2128) radius 1.25
  circle A483 centre (91.2857, 12.2128) radius 1.25
  circle A484 centre (95.75, 12.2128) radius 1.25
  circle A485 centre (100.2143, 12.2128) radius 1.25
  circle A486 centre (104.6786, 12.2128) radius 1.25
  circle A487 centre (109.1429, 12.2128) radius 1.25
  circle A488 centre (113.6071, 12.2128) radius 1.25
  circle A489 centre (118.0714, 12.2128) radius 1.25
  circle A490 centre (122.5357, 12.2128) radius 1.25
  circle A491 centre (127, 12.2128) radius 1.25
  circle A492 centre (42.1786, 17.3191) radius 1.25
  circle A493 centre (46.6429, 17.3191) radius 1.25
  circle A494 centre (51.1071, 17.3191) radius 1.25
  circle A495 centre (55.5714, 17.3191) radius 1.25
  circle A496 centre (60.0357, 17.3191) radius 1.25
  circle A497 centre (64.5, 17.3191) radius 1.25
  circle A498 centre (68.9643, 17.3191) radius 1.25
  circle A499 centre (73.4286, 17.3191) radius 1.25
  circle A500 centre (77.8929, 17.3191) radius 1.25
  circle A501 centre (82.3571, 17.3191) radius 1.25
  circle A502 centre (86.8214, 17.3191) radius 1.25
  circle A503 centre (91.2857, 17.3191) radius 1.25
  circle A504 centre (95.75, 17.3191) radius 1.25
  circle A505 centre (100.2143, 17.3191) radius 1.25
  circle A506 centre (104.6786, 17.3191) radius 1.25
  circle A507 centre (109.1429, 17.3191) radius 1.25
  circle A508 centre (113.6071, 17.3191) radius 1.25
  circle A509 centre (118.0714, 17.3191) radius 1.25
  circle A510 centre (122.5357, 17.3191) radius 1.25
  circle A511 centre (127, 17.3191) radius 1.25
  circle A512 centre (42.1786, 22.4255) radius 1.25
  circle A513 centre (46.6429, 22.4255) radius 1.25
  circle A514 centre (51.1071, 22.4255) radius 1.25
  circle A515 centre (55.5714, 22.4255) radius 1.25
  circle A516 centre (60.0357, 22.4255) radius 1.25
  circle A517 centre (64.5, 22.4255) radius 1.25
  circle A518 centre (68.9643, 22.4255) radius 1.25
  circle A519 centre (73.4286, 22.4255) radius 1.25
  circle A520 centre (77.8929, 22.4255) radius 1.25
  circle A521 centre (82.3571, 22.4255) radius 1.25
  circle A522 centre (86.8214, 22.4255) radius 1.25
  circle A523 centre (91.2857, 22.4255) radius 1.25
  circle A524 centre (95.75, 22.4255) radius 1.25
  circle A525 centre (100.2143, 22.4255) radius 1.25
  circle A526 centre (104.6786, 22.4255) radius 1.25
  circle A527 centre (109.1429, 22.4255) radius 1.25
  circle A528 centre (113.6071, 22.4255) radius 1.25
  circle A529 centre (118.0714, 22.4255) radius 1.25
  circle A530 centre (122.5357, 22.4255) radius 1.25
  circle A531 centre (127, 22.4255) radius 1.25
  circle A532 centre (42.1786, 27.5319) radius 1.25
  circle A533 centre (46.6429, 27.5319) radius 1.25
  circle A534 centre (51.1071, 27.5319) radius 1.25
  circle A535 centre (55.5714, 27.5319) radius 1.25
  circle A536 centre (60.0357, 27.5319) radius 1.25
  circle A537 centre (64.5, 27.5319) radius 1.25
  circle A538 centre (68.9643, 27.5319) radius 1.25
  circle A539 centre (73.4286, 27.5319) radius 1.25
  circle A540 centre (77.8929, 27.5319) radius 1.25
  circle A541 centre (82.3571, 27.5319) radius 1.25
  circle A542 centre (86.8214, 27.5319) radius 1.25
  circle A543 centre (91.2857, 27.5319) radius 1.25
  circle A544 centre (95.75, 27.5319) radius 1.25
  circle A545 centre (100.2143, 27.5319) radius 1.25
  circle A546 centre (104.6786, 27.5319) radius 1.25
  circle A547 centre (109.1429, 27.5319) radius 1.25
  circle A548 centre (113.6071, 27.5319) radius 1.25
  circle A549 centre (118.0714, 27.5319) radius 1.25
  circle A550 centre (122.5357, 27.5319) radius 1.25
  circle A551 centre (127, 27.5319) radius 1.25
  circle A552 centre (42.1786, 32.6383) radius 1.25
  circle A553 centre (46.6429, 32.6383) radius 1.25
  circle A554 centre (51.1071, 32.6383) radius 1.25
  circle A555 centre (55.5714, 32.6383) radius 1.25
  circle A556 centre (60.0357, 32.6383) radius 1.25
  circle A557 centre (64.5, 32.6383) radius 1.25
  circle A558 centre (68.9643, 32.6383) radius 1.25
  circle A559 centre (73.4286, 32.6383) radius 1.25
  circle A560 centre (77.8929, 32.6383) radius 1.25
  circle A561 centre (82.3571, 32.6383) radius 1.25
  circle A562 centre (86.8214, 32.6383) radius 1.25
  circle A563 centre (91.2857, 32.6383) radius 1.25
  circle A564 centre (95.75, 32.6383) radius 1.25
  circle A565 centre (100.2143, 32.6383) radius 1.25
  circle A566 centre (104.6786, 32.6383) radius 1.25
  circle A567 centre (109.1429, 32.6383) radius 1.25
  circle A568 centre (113.6071, 32.6383) radius 1.25
  circle A569 centre (118.0714, 32.6383) radius 1.25
  circle A570 centre (122.5357, 32.6383) radius 1.25
  circle A571 centre (127, 32.6383) radius 1.25
  circle A572 centre (42.1786, 37.7447) radius 1.25
  circle A573 centre (46.6429, 37.7447) radius 1.25
  circle A574 centre (51.1071, 37.7447) radius 1.25
  circle A575 centre (55.5714, 37.7447) radius 1.25
  circle A576 centre (60.0357, 37.7447) radius 1.25
  circle A577 centre (64.5, 37.7447) radius 1.25
  circle A578 centre (68.9643, 37.7447) radius 1.25
  circle A579 centre (73.4286, 37.7447) radius 1.25
  circle A580 centre (77.8929, 37.7447) radius 1.25
  circle A581 centre (82.3571, 37.7447) radius 1.25
  circle A582 centre (86.8214, 37.7447) radius 1.25
  circle A583 centre (91.2857, 37.7447) radius 1.25
  circle A584 centre (95.75, 37.7447) radius 1.25
  circle A585 centre (100.2143, 37.7447) radius 1.25
  circle A586 centre (104.6786, 37.7447) radius 1.25
  circle A587 centre (109.1429, 37.7447) radius 1.25
  circle A588 centre (113.6071, 37.7447) radius 1.25
  circle A589 centre (118.0714, 37.7447) radius 1.25
  circle A590 centre (122.5357, 37.7447) radius 1.25
  circle A591 centre (127, 37.7447) radius 1.25
  circle A592 centre (42.1786, 42.8511) radius 1.25
  circle A593 centre (46.6429, 42.8511) radius 1.25
  circle A594 centre (51.1071, 42.8511) radius 1.25
  circle A595 centre (55.5714, 42.8511) radius 1.25
  circle A596 centre (60.0357, 42.8511) radius 1.25
  circle A597 centre (64.5, 42.8511) radius 1.25
  circle A598 centre (68.9643, 42.8511) radius 1.25
  circle A599 centre (73.4286, 42.8511) radius 1.25
  circle A600 centre (77.8929, 42.8511) radius 1.25
  circle A601 centre (82.3571, 42.8511) radius 1.25
  circle A602 centre (86.8214, 42.8511) radius 1.25
  circle A603 centre (91.2857, 42.8511) radius 1.25
  circle A604 centre (95.75, 42.8511) radius 1.25
  circle A605 centre (100.2143, 42.8511) radius 1.25
  circle A606 centre (104.6786, 42.8511) radius 1.25
  circle A607 centre (109.1429, 42.8511) radius 1.25
  circle A608 centre (113.6071, 42.8511) radius 1.25
  circle A609 centre (118.0714, 42.8511) radius 1.25
  circle A610 centre (122.5357, 42.8511) radius 1.25
  circle A611 centre (127, 42.8511) radius 1.25
  circle A612 centre (42.1786, 47.9574) radius 1.25
  circle A613 centre (46.6429, 47.9574) radius 1.25
  circle A614 centre (51.1071, 47.9574) radius 1.25
  circle A615 centre (55.5714, 47.9574) radius 1.25
  circle A616 centre (60.0357, 47.9574) radius 1.25
  circle A617 centre (64.5, 47.9574) radius 1.25
  circle A618 centre (68.9643, 47.9574) radius 1.25
  circle A619 centre (73.4286, 47.9574) radius 1.25
  circle A620 centre (77.8929, 47.9574) radius 1.25
  circle A621 centre (82.3571, 47.9574) radius 1.25
  circle A622 centre (86.8214, 47.9574) radius 1.25
  circle A623 centre (91.2857, 47.9574) radius 1.25
  circle A624 centre (95.75, 47.9574) radius 1.25
  circle A625 centre (100.2143, 47.9574) radius 1.25
  circle A626 centre (104.6786, 47.9574) radius 1.25
  circle A627 centre (109.1429, 47.9574) radius 1.25
  circle A628 centre (113.6071, 47.9574) radius 1.25
  circle A629 centre (118.0714, 47.9574) radius 1.25
  circle A630 centre (122.5357, 47.9574) radius 1.25
  circle A631 centre (127, 47.9574) radius 1.25
  circle A632 centre (42.1786, 53.0638) radius 1.25
  circle A633 centre (46.6429, 53.0638) radius 1.25
  circle A634 centre (51.1071, 53.0638) radius 1.25
  circle A635 centre (55.5714, 53.0638) radius 1.25
  circle A636 centre (60.0357, 53.0638) radius 1.25
  circle A637 centre (64.5, 53.0638) radius 1.25
  circle A638 centre (68.9643, 53.0638) radius 1.25
  circle A639 centre (73.4286, 53.0638) radius 1.25
  circle A640 centre (77.8929, 53.0638) radius 1.25
  circle A641 centre (82.3571, 53.0638) radius 1.25
  circle A642 centre (86.8214, 53.0638) radius 1.25
  circle A643 centre (91.2857, 53.0638) radius 1.25
  circle A644 centre (95.75, 53.0638) radius 1.25
  circle A645 centre (100.2143, 53.0638) radius 1.25
  circle A646 centre (104.6786, 53.0638) radius 1.25
  circle A647 centre (109.1429, 53.0638) radius 1.25
  circle A648 centre (113.6071, 53.0638) radius 1.25
  circle A649 centre (118.0714, 53.0638) radius 1.25
  circle A650 centre (122.5357, 53.0638) radius 1.25
  circle A651 centre (127, 53.0638) radius 1.25
  circle A652 centre (42.1786, 58.1702) radius 1.25
  circle A653 centre (46.6429, 58.1702) radius 1.25
  circle A654 centre (51.1071, 58.1702) radius 1.25
  circle A655 centre (55.5714, 58.1702) radius 1.25
  circle A656 centre (60.0357, 58.1702) radius 1.25
  circle A657 centre (64.5, 58.1702) radius 1.25
  circle A658 centre (68.9643, 58.1702) radius 1.25
  circle A659 centre (73.4286, 58.1702) radius 1.25
  circle A660 centre (77.8929, 58.1702) radius 1.25
  circle A661 centre (82.3571, 58.1702) radius 1.25
  circle A662 centre (86.8214, 58.1702) radius 1.25
  circle A663 centre (91.2857, 58.1702) radius 1.25
  circle A664 centre (95.75, 58.1702) radius 1.25
  circle A665 centre (100.2143, 58.1702) radius 1.25
  circle A666 centre (104.6786, 58.1702) radius 1.25
  circle A667 centre (109.1429, 58.1702) radius 1.25
  circle A668 centre (113.6071, 58.1702) radius 1.25
  circle A669 centre (118.0714, 58.1702) radius 1.25
  circle A670 centre (122.5357, 58.1702) radius 1.25
  circle A671 centre (127, 58.1702) radius 1.25
  circle A672 centre (42.1786, 63.2766) radius 1.25
  circle A673 centre (46.6429, 63.2766) radius 1.25
  circle A674 centre (51.1071, 63.2766) radius 1.25
  circle A675 centre (55.5714, 63.2766) radius 1.25
  circle A676 centre (60.0357, 63.2766) radius 1.25
  circle A677 centre (64.5, 63.2766) radius 1.25
  circle A678 centre (68.9643, 63.2766) radius 1.25
  circle A679 centre (73.4286, 63.2766) radius 1.25
  circle A680 centre (77.8929, 63.2766) radius 1.25
  circle A681 centre (82.3571, 63.2766) radius 1.25
  circle A682 centre (86.8214, 63.2766) radius 1.25
  circle A683 centre (91.2857, 63.2766) radius 1.25
  circle A684 centre (95.75, 63.2766) radius 1.25
  circle A685 centre (100.2143, 63.2766) radius 1.25
  circle A686 centre (104.6786, 63.2766) radius 1.25
  circle A687 centre (109.1429, 63.2766) radius 1.25
  circle A688 centre (113.6071, 63.2766) radius 1.25
  circle A689 centre (118.0714, 63.2766) radius 1.25
  circle A690 centre (122.5357, 63.2766) radius 1.25
  circle A691 centre (127, 63.2766) radius 1.25
  circle A692 centre (42.1786, 68.383) radius 1.25
  circle A693 centre (46.6429, 68.383) radius 1.25
  circle A694 centre (51.1071, 68.383) radius 1.25
  circle A695 centre (55.5714, 68.383) radius 1.25
  circle A696 centre (60.0357, 68.383) radius 1.25
  circle A697 centre (64.5, 68.383) radius 1.25
  circle A698 centre (68.9643, 68.383) radius 1.25
  circle A699 centre (73.4286, 68.383) radius 1.25
  circle A700 centre (77.8929, 68.383) radius 1.25
  circle A701 centre (82.3571, 68.383) radius 1.25
  circle A702 centre (86.8214, 68.383) radius 1.25
  circle A703 centre (91.2857, 68.383) radius 1.25
  circle A704 centre (95.75, 68.383) radius 1.25
  circle A705 centre (100.2143, 68.383) radius 1.25
  circle A706 centre (104.6786, 68.383) radius 1.25
  circle A707 centre (109.1429, 68.383) radius 1.25
  circle A708 centre (113.6071, 68.383) radius 1.25
  circle A709 centre (118.0714, 68.383) radius 1.25
  circle A710 centre (122.5357, 68.383) radius 1.25
  circle A711 centre (127, 68.383) radius 1.25
  circle A712 centre (42.1786, 73.4894) radius 1.25
  circle A713 centre (46.6429, 73.4894) radius 1.25
  circle A714 centre (51.1071, 73.4894) radius 1.25
  circle A715 centre (55.5714, 73.4894) radius 1.25
  circle A716 centre (60.0357, 73.4894) radius 1.25
  circle A717 centre (64.5, 73.4894) radius 1.25
  circle A718 centre (68.9643, 73.4894) radius 1.25
  circle A719 centre (73.4286, 73.4894) radius 1.25
  circle A720 centre (77.8929, 73.4894) radius 1.25
  circle A721 centre (82.3571, 73.4894) radius 1.25
  circle A722 centre (86.8214, 73.4894) radius 1.25
  circle A723 centre (91.2857, 73.4894) radius 1.25
  circle A724 centre (95.75, 73.4894) radius 1.25
  circle A725 centre (100.2143, 73.4894) radius 1.25
  circle A726 centre (104.6786, 73.4894) radius 1.25
  circle A727 centre (109.1429, 73.4894) radius 1.25
  circle A728 centre (113.6071, 73.4894) radius 1.25
  circle A729 centre (118.0714, 73.4894) radius 1.25
  circle A730 centre (122.5357, 73.4894) radius 1.25
  circle A731 centre (127, 73.4894) radius 1.25
  circle A732 centre (42.1786, 78.5957) radius 1.25
  circle A733 centre (46.6429, 78.5957) radius 1.25
  circle A734 centre (51.1071, 78.5957) radius 1.25
  circle A735 centre (55.5714, 78.5957) radius 1.25
  circle A736 centre (60.0357, 78.5957) radius 1.25
  circle A737 centre (64.5, 78.5957) radius 1.25
  circle A738 centre (68.9643, 78.5957) radius 1.25
  circle A739 centre (73.4286, 78.5957) radius 1.25
  circle A740 centre (77.8929, 78.5957) radius 1.25
  circle A741 centre (82.3571, 78.5957) radius 1.25
  circle A742 centre (86.8214, 78.5957) radius 1.25
  circle A743 centre (91.2857, 78.5957) radius 1.25
  circle A744 centre (95.75, 78.5957) radius 1.25
  circle A745 centre (100.2143, 78.5957) radius 1.25
  circle A746 centre (104.6786, 78.5957) radius 1.25
  circle A747 centre (109.1429, 78.5957) radius 1.25
  circle A748 centre (113.6071, 78.5957) radius 1.25
  circle A749 centre (118.0714, 78.5957) radius 1.25
  circle A750 centre (122.5357, 78.5957) radius 1.25
  circle A751 centre (127, 78.5957) radius 1.25
  circle A752 centre (42.1786, 83.7021) radius 1.25
  circle A753 centre (46.6429, 83.7021) radius 1.25
  circle A754 centre (51.1071, 83.7021) radius 1.25
  circle A755 centre (55.5714, 83.7021) radius 1.25
  circle A756 centre (60.0357, 83.7021) radius 1.25
  circle A757 centre (64.5, 83.7021) radius 1.25
  circle A758 centre (68.9643, 83.7021) radius 1.25
  circle A759 centre (73.4286, 83.7021) radius 1.25
  circle A760 centre (77.8929, 83.7021) radius 1.25
  circle A761 centre (82.3571, 83.7021) radius 1.25
  circle A762 centre (86.8214, 83.7021) radius 1.25
  circle A763 centre (91.2857, 83.7021) radius 1.25
  circle A764 centre (95.75, 83.7021) radius 1.25
  circle A765 centre (100.2143, 83.7021) radius 1.25
  circle A766 centre (104.6786, 83.7021) radius 1.25
  circle A767 centre (109.1429, 83.7021) radius 1.25
  circle A768 centre (113.6071, 83.7021) radius 1.25
  circle A769 centre (118.0714, 83.7021) radius 1.25
  circle A770 centre (122.5357, 83.7021) radius 1.25
  circle A771 centre (127, 83.7021) radius 1.25
  circle A772 centre (42.1786, 88.8085) radius 1.25
  circle A773 centre (46.6429, 88.8085) radius 1.25
  circle A774 centre (51.1071, 88.8085) radius 1.25
  circle A775 centre (55.5714, 88.8085) radius 1.25
  circle A776 centre (60.0357, 88.8085) radius 1.25
  circle A777 centre (64.5, 88.8085) radius 1.25
  circle A778 centre (68.9643, 88.8085) radius 1.25
  circle A779 centre (73.4286, 88.8085) radius 1.25
  circle A780 centre (77.8929, 88.8085) radius 1.25
  circle A781 centre (82.3571, 88.8085) radius 1.25
  circle A782 centre (86.8214, 88.8085) radius 1.25
  circle A783 centre (91.2857, 88.8085) radius 1.25
  circle A784 centre (95.75, 88.8085) radius 1.25
  circle A785 centre (100.2143, 88.8085) radius 1.25
  circle A786 centre (104.6786, 88.8085) radius 1.25
  circle A787 centre (109.1429, 88.8085) radius 1.25
  circle A788 centre (113.6071, 88.8085) radius 1.25
  circle A789 centre (118.0714, 88.8085) radius 1.25
  circle A790 centre (122.5357, 88.8085) radius 1.25
  circle A791 centre (127, 88.8085) radius 1.25
  circle A792 centre (42.1786, 93.9149) radius 1.25
  circle A793 centre (46.6429, 93.9149) radius 1.25
  circle A794 centre (51.1071, 93.9149) radius 1.25
  circle A795 centre (55.5714, 93.9149) radius 1.25
  circle A796 centre (60.0357, 93.9149) radius 1.25
  circle A797 centre (64.5, 93.9149) radius 1.25
  circle A798 centre (68.9643, 93.9149) radius 1.25
  circle A799 centre (73.4286, 93.9149) radius 1.25
  circle A800 centre (77.8929, 93.9149) radius 1.25
  circle A801 centre (82.3571, 93.9149) radius 1.25
  circle A802 centre (86.8214, 93.9149) radius 1.25
  circle A803 centre (91.2857, 93.9149) radius 1.25
  circle A804 centre (95.75, 93.9149) radius 1.25